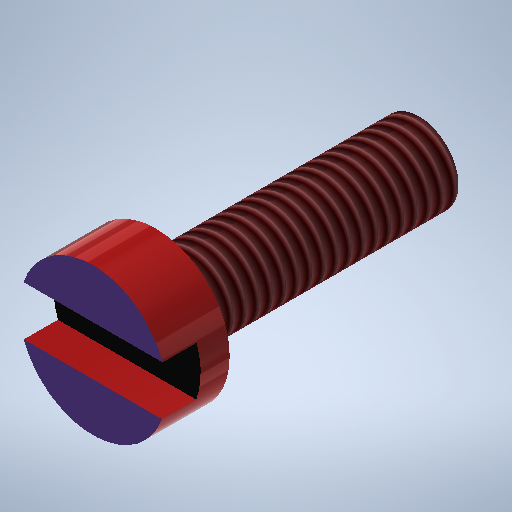
# Autodesk Inventor part: Parafuso-M3-5
Saved by Autodesk Inventor 2025 (Build 290162000, 162)
## iProperties
Created: 2016-06-24
Part Number: Parafuso-M3-5
Material: Genérico
Document SubType Name: Modeling
Designer: MarceloAdmin
Density: 1 g/cm^3
Appearance: Suave - Vermelho
Author: MarceloAdmin
Autodesk Inventor part; units mm, degrees
ref_plane "YZ Plane" through (0, 0, 0) normal (1, 0, 0) x (0, 1, 0)
ref_plane "XZ Plane" through (0, 0, 0) normal (0, 1, 0) x (-1, 0, 0)
ref_plane "XY Plane" through (0, 0, 0) normal (0, 0, 1) x (1, 0, 0)
sketch "Esboço1" plane through (0, 0, 0) normal (0, 1, 0) x (-1, 0, 0)
  circle A0 centre (0, 0) radius 2.8
  dimension "d0" = 5.6
  constraints: 1 centre point, 1 coincident
  measures "d0" diameter of A0
extrude "Extrusão1" add sketch "Esboço1" along normal blind 2.4
sketch "Esboço2" plane through (0, 0, 0) normal (1, 0, 0) x (0, 1, 0)
  line L0 (0, 0.9185) -> (1.2961, 0.9185)
  line L1 (1.2961, 0.9185) -> (1.2961, -0.9611)
  line L2 (1.2961, -0.9611) -> (0, -0.9611)
  line L3 (0, -0.9611) -> (0, 0.9185)
  point P0 (0, 0)
  constraints: 8 end point, 2 parallel, 1 horizontal, 1 perpendicular
extrude "Extrusão2" cut sketch "Esboço2" along normal through all both and the other way through all
sketch "Esboço3" plane through (0, 2.4, 0) normal (0, 1, 0) x (1, 0, 0)
  circle A0 centre (0, 0) radius 2.8 projected
  circle A1 centre (0, 0) radius 1.5
  dimension "d5" = 3
  constraints: 1 centre point, 1 coincident
  measures "d5" diameter of A1
extrude "Extrusão3" add sketch "Esboço3" along normal blind 10 contours A1
thread "Rosca1" size "M3x0.5" class "6g" standard "ANSI Metric M Profile" full length
